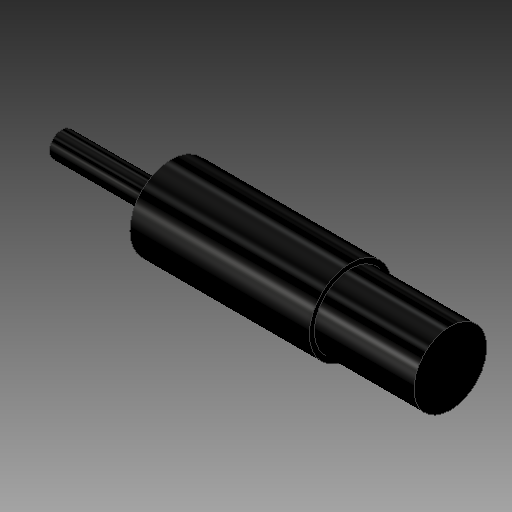
# Autodesk Inventor part: Circuit_PhonePlug_MP-101MH
Saved by Autodesk Inventor 2018.2 (Build 222227000, 227)
## iProperties
Created: 2018-02-16
Part Number: Circuit_PhonePlug_MP-101MH
Material: ABS プラスチック
Document SubType Name: Modeling
Designer: sktom
Density: 1.06 g/cm^3
Appearance: 黒
Author: sktom
Title: Circuit_PhonePlug_MP-101MH
Autodesk Inventor part; units mm, degrees
ref_plane "YZ Plane" through (0, 0, 0) normal (1, 0, 0) x (0, 1, 0)
ref_plane "XZ Plane" through (0, 0, 0) normal (0, 1, 0) x (-1, 0, 0)
ref_plane "XY Plane" through (0, 0, 0) normal (0, 0, 1) x (1, 0, 0)
sketch "スケッチ1" plane through (0, 0, 0) normal (0, 0, 1) x (1, 0, 0)
  line L0 (0, 0) -> (0, 1.25)
  line L1 (0, 1.25) -> (11, 1.25)
  line L2 (11, 1.25) -> (11, 4.15)
  line L3 (11, 4.15) -> (29, 4.15)
  line L4 (29, 4.15) -> (29, 3.65)
  line L5 (29, 3.65) -> (39, 3.65)
  line L6 (39, 3.65) -> (39, 0)
  line L7 (39, 0) -> (0, 0)
  dimension "d0" = 1.25
  dimension "d1" = 11
  dimension "d2" = 18
  dimension "d3" = 4.15
  dimension "d4" = 0.5
  dimension "d5" = 10
  constraints: 16 end point, 7 perpendicular, 1 vertical
  measures "d0" distance between parallel lines of L7 L1
  measures "d1" distance of L0.end L1.end
  measures "d2" distance of L2.end L3.end
  measures "d3" distance between parallel lines of L7 L3
  measures "d4" distance between parallel lines of L3 L5
  measures "d5" distance of L4.end L5.end
revolve "回転1" add sketch "スケッチ1" angle 360 about axis through (39, 0, 0) along (-1, 0, 0)
